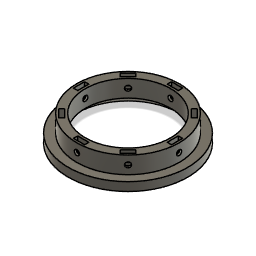
couplage_standard_male v8 (Autodesk Fusion 360 design; units mm, degrees)
Autodesk Fusion 360 part; units mm, degrees
sketch "Esquisse1" plane through (0, 0, 0) normal (0, 1, 0) x (1, 0, 0)
  circle A0 centre (0, 0) radius 30
  circle A1 centre (0, 0) radius 25
  dimension "d1" = 60
  constraint coincident A0.centre A1.centre
  constraint concentric A0 A1
  measures "d1" diameter of A0
extrude "Extrusion1" add sketch "Esquisse1" along normal mid plane 10
sketch "Esquisse2" plane through (0, -5, 0) normal (0, -1, 0) x (1, 0, 0)
  circle A0 centre (0, 0) radius 25
  circle A1 centre (0, 0) radius 30
  circle A2 centre (0, 0) radius 35
  dimension "d4" = 70
  constraint coincident A0.centre A1.centre
  measures "d4" diameter of A2
extrude "Extrusion2" add sketch "Esquisse2" along normal blind 5 contours A1 | A2
ref_plane "Plan de construction1" through (30, 0, 0) normal (1, 0, 0) x (0, 1, 0)
ref_plane "Plan de construction2" through (-30, 0, 0) normal (1, 0, 0) x (0, 1, 0)
ref_plane "Plan de construction3" through (0, 0, 30) normal (0, 0, 1) x (1, 0, 0)
ref_plane "Plan de construction4" through (0, 0, -30) normal (0, 0, 1) x (1, 0, 0)
sketch "Esquisse3" plane through (30, 0, 0) normal (1, 0, 0) x (0, 0, -1)
  circle A0 centre (0, 0) radius 1.5
  dimension "d11" = 3
  constraint coincident A0.centre origin
  measures "d11" diameter of A0
extrude "Extrusion3" cut sketch "Esquisse3" against normal blind 60
sketch "Esquisse4" plane through (0, 0, -30) normal (0, 0, 1) x (1, 0, 0)
  circle A0 centre (0, 0) radius 1.5
  dimension "d14" = 3
  constraint coincident A0.centre origin
  measures "d14" diameter of A0
extrude "Extrusion4" cut sketch "Esquisse4" along normal blind 60
sketch "Esquisse5" plane through (0, 5, 0) normal (0, 1, 0) x (-1, 0, 0)
  circle A0 centre (0, 0) radius 25
  circle A1 centre (0, 0) radius 30
  line L0 (0, 30) -> (0, 25) construction
  line L1 (0, 27.5) -> (-5, 27.5) construction
  line L2 (0, 27.5) -> (5, 27.5) construction
  line L3 (0, 27.5) -> (0, 26.25)
  line L4 (0, 27.5) -> (0, 28.75)
  line L5 (0, 26.25) -> (3.25, 26.25)
  line L6 (0, 28.75) -> (3.25, 28.75)
  line L7 (3.25, 28.75) -> (3.25, 26.25)
  line L8 (0, 26.25) -> (-3.25, 26.25)
  line L9 (0, 28.75) -> (-3.25, 28.75)
  line L10 (-3.25, 28.75) -> (-3.25, 26.25)
  line L11 (-18.5616, 18.5616) -> (-16.2635, 20.8597)
  line L12 (-19.4454, 19.4454) -> (-18.5616, 18.5616)
  line L13 (-19.4454, 19.4454) -> (-20.3293, 20.3293)
  line L14 (-20.3293, 20.3293) -> (-18.0312, 22.6274)
  line L15 (-18.0312, 22.6274) -> (-16.2635, 20.8597)
  line L16 (-18.5616, 18.5616) -> (-20.8597, 16.2635)
  line L17 (-22.6274, 18.0312) -> (-20.8597, 16.2635)
  line L18 (-20.3293, 20.3293) -> (-22.6274, 18.0312)
  line L19 (-19.4454, 19.4454) -> (-22.981, 15.9099) construction
  line L20 (-19.4454, 19.4454) -> (-15.9099, 22.981) construction
  line L21 (-21.2132, 21.2132) -> (-17.6777, 17.6777) construction
  line L22 (-26.25, 0) -> (-26.25, 3.25)
  line L23 (-27.5, 0) -> (-26.25, 0)
  line L24 (-27.5, 0) -> (-28.75, 0)
  line L25 (-28.75, 0) -> (-28.75, 3.25)
  line L26 (-28.75, 3.25) -> (-26.25, 3.25)
  line L27 (-26.25, 0) -> (-26.25, -3.25)
  line L28 (-28.75, -3.25) -> (-26.25, -3.25)
  line L29 (-28.75, 0) -> (-28.75, -3.25)
  line L30 (-27.5, 0) -> (-27.5, -5) construction
  line L31 (-27.5, 0) -> (-27.5, 5) construction
  line L32 (-30, 0) -> (-25, 0) construction
  line L33 (-18.5616, -18.5616) -> (-20.8597, -16.2635)
  line L34 (-19.4454, -19.4454) -> (-18.5616, -18.5616)
  line L35 (-19.4454, -19.4454) -> (-20.3293, -20.3293)
  line L36 (-20.3293, -20.3293) -> (-22.6274, -18.0312)
  line L37 (-22.6274, -18.0312) -> (-20.8597, -16.2635)
  line L38 (-18.5616, -18.5616) -> (-16.2635, -20.8597)
  line L39 (-18.0312, -22.6274) -> (-16.2635, -20.8597)
  line L40 (-20.3293, -20.3293) -> (-18.0312, -22.6274)
  line L41 (-19.4454, -19.4454) -> (-15.9099, -22.981) construction
  line L42 (-19.4454, -19.4454) -> (-22.981, -15.9099) construction
  line L43 (-21.2132, -21.2132) -> (-17.6777, -17.6777) construction
  line L44 (0, -26.25) -> (-3.25, -26.25)
  line L45 (0, -27.5) -> (0, -26.25)
  line L46 (0, -27.5) -> (0, -28.75)
  line L47 (0, -28.75) -> (-3.25, -28.75)
  line L48 (-3.25, -28.75) -> (-3.25, -26.25)
  line L49 (0, -26.25) -> (3.25, -26.25)
  line L50 (3.25, -28.75) -> (3.25, -26.25)
  line L51 (0, -28.75) -> (3.25, -28.75)
  line L52 (0, -27.5) -> (5, -27.5) construction
  line L53 (0, -27.5) -> (-5, -27.5) construction
  line L54 (0, -30) -> (0, -25) construction
  line L55 (18.5616, -18.5616) -> (16.2635, -20.8597)
  line L56 (19.4454, -19.4454) -> (18.5616, -18.5616)
  line L57 (19.4454, -19.4454) -> (20.3293, -20.3293)
  line L58 (20.3293, -20.3293) -> (18.0312, -22.6274)
  line L59 (18.0312, -22.6274) -> (16.2635, -20.8597)
  line L60 (18.5616, -18.5616) -> (20.8597, -16.2635)
  line L61 (22.6274, -18.0312) -> (20.8597, -16.2635)
  line L62 (20.3293, -20.3293) -> (22.6274, -18.0312)
  line L63 (19.4454, -19.4454) -> (22.981, -15.9099) construction
  line L64 (19.4454, -19.4454) -> (15.9099, -22.981) construction
  line L65 (21.2132, -21.2132) -> (17.6777, -17.6777) construction
  line L66 (26.25, 0) -> (26.25, -3.25)
  line L67 (27.5, 0) -> (26.25, 0)
  line L68 (27.5, 0) -> (28.75, 0)
  line L69 (28.75, 0) -> (28.75, -3.25)
  line L70 (28.75, -3.25) -> (26.25, -3.25)
  line L71 (26.25, 0) -> (26.25, 3.25)
  line L72 (28.75, 3.25) -> (26.25, 3.25)
  line L73 (28.75, 0) -> (28.75, 3.25)
  line L74 (27.5, 0) -> (27.5, 5) construction
  line L75 (27.5, 0) -> (27.5, -5) construction
  line L76 (30, 0) -> (25, 0) construction
  line L77 (18.5616, 18.5616) -> (20.8597, 16.2635)
  line L78 (19.4454, 19.4454) -> (18.5616, 18.5616)
  line L79 (19.4454, 19.4454) -> (20.3293, 20.3293)
  line L80 (20.3293, 20.3293) -> (22.6274, 18.0312)
  line L81 (22.6274, 18.0312) -> (20.8597, 16.2635)
  line L82 (18.5616, 18.5616) -> (16.2635, 20.8597)
  line L83 (18.0312, 22.6274) -> (16.2635, 20.8597)
  line L84 (20.3293, 20.3293) -> (18.0312, 22.6274)
  line L85 (19.4454, 19.4454) -> (15.9099, 22.981) construction
  line L86 (19.4454, 19.4454) -> (22.981, 15.9099) construction
  line L87 (21.2132, 21.2132) -> (17.6777, 17.6777) construction
  dimension "d17" = 1.25
  dimension "d18" = 1.25
  dimension "d19" = 3.25
  dimension "d20" = 3.25
  dimension "d21" = 3.25
  dimension "d25" = 360
  constraint coincident A1 L0.start
  constraint coincident A0 L0.end
  constraint vertical L0
  constraint midpoint L0 L1.start
  constraint perpendicular L0 L1
  constraint perpendicular L0 L2
  constraint coincident L0 L3.end
  constraint perpendicular L1 L4
  constraint perpendicular L3 L5
  constraint perpendicular L4 L6
  constraint perpendicular L3 L8
  constraint perpendicular L0 L9
  constraint perpendicular L8 L10
  measures "d17" distance of L1.start L3.end
  measures "d18" distance of L1.start L4.end
  measures "d19" distance of L3.end L5.end
  measures "d20" distance of L4.end L6.end
  measures "d21" distance of L3.end L8.end
extrude "Extrusion6" cut sketch "Esquisse5" against normal blind 8 contours L3 L4 L5 L6 L7 | L3 L4 L8 L9 L10 | L11 L12 L13 L14 L15 | L12 L13 L16 L17 L18 | L22 L23 L24 L25 L26 | L23 L24 L27 L28 L29 | L33 L34 L35 L36 L37 | L34 L35 L38 L39 L40 | L44 L45 L46 L47 L48 | L45 L46 L49 L50 L51 | L55 L56 L57 L58 L59 | L56 L57 L60 L61 L62 | L66 L67 L68 L69 L70 | L67 L68 L71 L72 L73 | L77 L78 L79 L80 L81 | L78 L79 L82 L83 L84
move_body "Déplacer1" bodies 1 to x (0.707107, 0, 0.707107) y (0, 1, 0) z (-0.707107, 0, 0.707107) at (0, 0, 0)
ref_plane "Plan de construction5" through (0, 0, -30) normal (0, 0, 1) x (1, 0, 0)
ref_plane "Plan de construction6" through (30, 0, 0) normal (1, 0, 0) x (0, 1, 0)
sketch "Esquisse6" plane through (30, 0, 0) normal (1, 0, 0) x (0, 0, -1)
  circle A0 centre (0, 0) radius 1.5
  dimension "d30" = 3
  constraint coincident A0.centre origin
  measures "d30" diameter of A0
sketch "Esquisse7" plane through (0, 0, -30) normal (0, 0, 1) x (1, 0, 0)
  circle A0 centre (0, 0) radius 1.5
  dimension "d31" = 3
  constraint coincident A0.centre origin
  measures "d31" diameter of A0
extrude "Extrusion7" cut sketch "Esquisse6" against normal blind 60
extrude "Extrusion8" cut sketch "Esquisse7" along normal blind 60
chamfer "Chanfrein1" distance 5 angle 45 1 edges at (-22.8739, -10, -10.0889)
equation "d17 = ( 2.5 / 2 ) * 1 mm"
equation "d18 = ( 2.5 / 2 ) * 1 mm"
equation "d19 = ( 6.5 / 2 ) * 1 mm"
equation "d20 = ( 6.5 / 2 ) * 1 mm"
equation "d21 = ( 6.5 / 2 ) * 1 mm"
